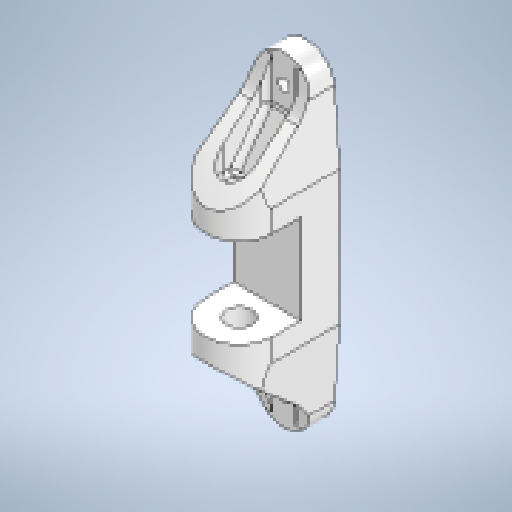
# Autodesk Inventor part: Bracket
Saved by Autodesk Inventor 2023.2 (Build 272271000, 271)
## iProperties
Created: 2022-05-26
Part Number: Bracket
Material: Nylon 6/6
Document SubType Name: Modeling
Designer: Nathan Cai
Density: 1.13472 g/cm^3
Appearance: Smooth - White
Mass: 16.25 g
Surface Area: 87.562 cm^2
Volume: 26.6495 cm^3
Author: Nathan Cai
Autodesk Inventor part; units mm, degrees
ref_plane "YZ Plane" through (0, 0, 0) normal (1, 0, 0) x (0, 1, 0)
ref_plane "XZ Plane" through (0, 0, 0) normal (0, 1, 0) x (-1, 0, 0)
ref_plane "XY Plane" through (0, 0, 0) normal (0, 0, 1) x (1, 0, 0)
sketch "Sketch15" plane through (0, 0, 0) normal (0, 0, 1) x (1, 0, 0)
  line L0 (0, 0) -> (19.05, 0)
  line L1 (19.05, 0) -> (19.05, 19.05)
  line L2 (19.05, 19.05) -> (0, 19.05)
  line L3 (0, 19.05) -> (0, 0)
  line L4 (9.525, 19.05) -> (9.525, 0) construction
  circle A0 centre (9.525, 38.1) radius 1.7526
  circle A1 centre (9.525, 38.1) radius 7.9375
  line L5 (0, 19.05) -> (1.614011, 38.748203)
  line L6 (17.435989, 38.748203) -> (19.05, 19.05)
  dimension "d79" = 19.05
  dimension "d80" = 19.05
  dimension "d81" = 3.5052
  dimension "d83" = 15.875
  dimension "d84" = 38.1
  constraints: 14 end point, 2 centre point, 2 midpoint, 2 parallel, 2 point on circle, 2 tangent, 1 coincident, 1 horizontal, 1 perpendicular, 1 point on line
  measures "d79" distance of L2.end L1.end
  measures "d80" distance of L1.end L0.end
  measures "d81" diameter of A0
  measures "d83" diameter of A1
  measures "d84" distance from line of L0 A0.centre
extrude "Extrusion12" add sketch "Sketch15" along normal blind 6.35
sketch "Sketch16" plane through (0, 0, 6.35) normal (0, 0, 1) x (1, 0, 0)
  line L0 (0, 19.05) -> (0, 0) projected
  line L1 (19.05, 0) -> (19.05, 19.05) projected
  line L2 (0, 19.05) -> (19.05, 19.05)
  line L3 (19.05, 19.05) -> (19.05, 12.7)
  line L4 (19.05, 12.7) -> (0, 12.7)
  line L5 (0, 12.7) -> (0, 19.05)
  dimension "d87" = 6.35
  constraints: 8 end point, 2 parallel, 1 horizontal, 1 perpendicular, 1 point on line
  measures "d87" distance of L2.end L3.end
extrude "Extrusion13" add sketch "Sketch16" along normal blind 22.225
fillet "Fillet15" radius 9.525 2 edges at (19.05, 15.875, 28.575) (0, 15.875, 28.575)
sketch "Sketch17" plane through (0, 19.05, 6.35) normal (0, 1, 0) x (1, 0, 0)
  arc A0 (0, -12.7) -> (19.05, -12.7) centre (9.525, -12.7) ccw projected
  circle A1 centre (9.525, -12.7) radius 3.683
  point P0 (0, 6.35)
  dimension "d91" = 7.366
  constraints: 1 centre point, 1 coincident
  measures "d91" diameter of A1
extrude "Extrusion14" cut sketch "Sketch17" against normal through all
sketch "Sketch18" plane through (0, 19.05, 6.35) normal (0, 1, 0) x (1, 0, 0)
  circle A0 centre (9.525, -12.7) radius 3.683 construction
  arc A1 (0, -12.7) -> (19.05, -12.7) centre (9.525, -12.7) ccw
  line L0 (0, 0) -> (0, -12.7) projected
  arc A2 (0, -12.7) -> (19.05, -12.7) centre (9.525, -12.7) ccw projected
  line L1 (0, -12.7) -> (19.05, -12.7) construction
  line L2 (13.208, -12.7) -> (6.858, -12.7) construction
  arc A3 (4.7625, -12.7) -> (14.2875, -12.7) centre (9.525, -12.7) ccw
  line L3 (19.05, 0) -> (19.05, -12.7)
  line L4 (19.05, -12.7) -> (0, -12.7) construction
  line L5 (0, -12.7) -> (0, 0)
  line L6 (14.2875, 0) -> (14.2875, -12.7)
  line L7 (14.2875, -12.7) -> (4.7625, -12.7) construction
  line L8 (4.7625, -12.7) -> (4.7625, 0)
  line L9 (0, 0) -> (4.7625, 0)
  line L10 (14.2875, 0) -> (19.05, 0)
  point P0 (0, 6.35)
  point P1 (12.7, 0.000461)
  point P2 (4.7625, -12.7)
  dimension "d96" = 4.7625
  constraints: 20 end point, 4 parallel, 4 point on circle, 4 point on line, 3 horizontal, 2 centre point, 2 coincident, 2 perpendicular, 2 tangent, 1 horizontal alignment, 1 other
  measures "d96" radius of A3
sketch "Sketch19" plane through (0, 0, 6.35) normal (0, 0, 1) x (1, 0, 0)
  circle A0 centre (9.525, 38.1) radius 1.7526
  arc A1 (14.2875, 38.1) -> (4.7625, 38.1) centre (9.525, 38.1) ccw
  line L0 (14.2875, 19.05) -> (14.2875, 38.1)
  line L1 (17.4891, 38.1) -> (1.5609, 38.1)
  line L2 (4.7625, 38.1) -> (4.7625, 19.05)
  line L3 (1.614011, 38.748203) -> (0, 19.05)
  line L4 (0, 19.05) -> (1.614011, 38.748203)
  arc A2 (17.435989, 38.748203) -> (1.614011, 38.748203) centre (9.525, 38.1) ccw
  line L5 (19.05, 19.05) -> (17.435989, 38.748203)
  arc A3 (17.435989, 38.748203) -> (1.614011, 38.748203) centre (9.525, 38.1) ccw
  line L6 (0, 0) -> (19.05, 0)
  line L7 (1.614011, 38.748203) -> (0, 19.05)
  line L8 (0, 19.05) -> (4.7625, 19.05)
  line L9 (0, 19.05) -> (19.05, 19.05)
  line L10 (14.2875, 19.05) -> (19.05, 19.05)
  line L11 (4.7625, 19.05) -> (14.2875, 19.05)
  line L12 (14.2875, 19.05) -> (14.2875, 25.4)
  line L13 (14.2875, 25.4) -> (4.7625, 25.4)
  line L14 (4.7625, 25.4) -> (4.7625, 19.05)
  point P0 (12.7, 19.05)
  dimension "d97" = 9.525
  dimension "d102" = 6.35
  constraints: 23 end point, 5 point on circle, 5 point on line, 4 parallel, 4 tangent, 2 centre point, 2 coincident, 2 collinear, 1 horizontal, 1 perpendicular
  measures "d97" diameter of A1
  measures "d102" distance of L12.end L11.end
ref_plane "Work Plane2" through (9.525, 0, 0) normal (1, 0, 0) x (0, 0, -1)
extrude "Extrusion16" add sketch "Sketch18" along normal blind 19.05
sketch "Sketch21" plane through (0, 0, 0) normal (0, 0, -1) x (-1, 0, 0)
  line L0 (-19.05, 19.05) -> (-17.435989, 38.748203)
  line L1 (-19.05, 19.05) -> (0, 19.05) construction
  line L2 (0, 19.05) -> (0, 38.1)
  line L3 (0, 38.1) -> (-19.05, 38.1)
  line L4 (-19.05, 38.1) -> (-19.05, 19.05)
  line L5 (-19.05, 19.05) -> (-17.4891, 38.1)
  line L6 (-1.614011, 38.748203) -> (0, 19.05)
  line L7 (0, 19.05) -> (-1.5609, 38.1)
  point P0 (0, 0)
  constraints: 12 end point, 4 point on line, 2 parallel, 1 horizontal, 1 perpendicular
extrude "Extrusion17" cut sketch "Sketch21" against normal through all
sketch "Sketch22" plane through (19.05, 0, 0) normal (1, 0, 0) x (0, 0, -1)
  line L0 (-28.575, 12.7) -> (-28.575, 38.1)
  line L1 (-6.35, 19.05) -> (-6.35, 38.1) construction
  line L2 (-28.575, 38.1) -> (-6.35, 38.1)
  line L3 (-6.35, 38.1) -> (-6.35, 19.05)
  line L4 (-6.35, 19.05) -> (-28.575, 19.05)
  line L5 (-28.575, 19.05) -> (-28.575, 38.1)
  line L6 (-6.35, 38.1) -> (-6.35, 38.748203)
  line L7 (-28.575, 19.05) -> (-6.35, 38.1)
  point P0 (0, 0)
  point P1 (-6.35, 38.1)
  dimension "d107" = 19.05
  constraints: 10 end point, 2 parallel, 1 horizontal, 1 perpendicular, 1 point on line
  measures "d107" distance between parallel lines of L4 L2
extrude "Extrusion18" cut sketch "Sketch22" against normal through all contours L0 L2 L7
fillet "Fillet16" radius 12.7 2 edges at (3.1617, 38.1, 6.35) (15.8883, 38.1, 6.35)
sketch "Sketch23" plane through (0, 0, 6.35) normal (0, 0, 1) x (1, 0, 0)
  circle A0 centre (9.525, 38.1) radius 1.7526 projected
  circle A1 centre (9.525, 38.1) radius 4.7625
  point P0 (0, 0)
  dimension "d112" = 9.525
  constraints: 1 centre point, 1 coincident
  measures "d112" diameter of A1
extrude "Extrusion19" cut sketch "Sketch23" along normal through all
chamfer "Chamfer2" distance 12.7 distance2 7.9375 1 edges at (9.525, 19.05, 6.35) measured on face at (9.525, 19.55, 6.35)
fillet "Fillet18" radius 1.5875 9 edges at (14.2875, 37.8456, 6.35) (4.7625, 37.8456, 6.35) (9.525, 19.05, 23.8125) (14.2875, 19.05, 16.6687) (4.7625, 19.05, 16.6687) (14.2875, 25.4, 10.3187) (4.7625, 25.4, 10.3187) (9.525, 31.75, 6.35) (9.525, 19.05, 14.2875)
mirror "Mirror4" about plane through (0, 0, 0) normal (0, -1, 0) of "Extrusion12", "Extrusion13", "Fillet15", "Extrusion14", "Extrusion16", "Extrusion17", "Extrusion18", "Fillet16", "Extrusion19", "Fillet18", "Chamfer2"
thicken "Thicken2" operation add thickness 4.7625 both sides no extend neighbours no toward (0, 0, 1) faces at (6.35, -4.233333, 6.35)
ref_plane "Work Plane3" through (9.525, 0, 0) normal (-1, 0, 0) x (0, 0, -1)
body "Solid3"
